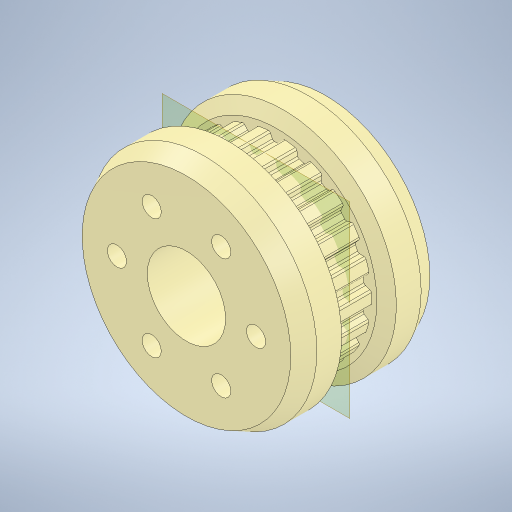
# Autodesk Inventor part: XL Pulley Generator
Saved by Autodesk Inventor 2023.4 (Build 274418000, 418)
## iProperties
RuleStatus: InUse
Created: 2022-06-22
Part Number: XL Pulley Generator
Material: Nylon 6/6
Document SubType Name: Modeling
Designer: Nathan Cai
Density: 1.13 g/cm^3
Appearance: Nylon 6
Mass: 3.49489 g
Surface Area: 67.8029 cm^2
Volume: 3.75794 cm^3
Author: Nathan Cai
Autodesk Inventor part; units mm, degrees
ref_plane "YZ Plane" through (0, 0, 0) normal (1, 0, 0) x (0, 1, 0)
ref_plane "XZ Plane" through (0, 0, 0) normal (0, 1, 0) x (-1, 0, 0)
ref_plane "XY Plane" through (0, 0, 0) normal (0, 0, 1) x (1, 0, 0)
sketch "Sketch2" plane through (0, 0, 0) normal (0, 0, 1) x (1, 0, 0)
  circle A0 centre (0, 0) radius 17.7872 construction
  circle A1 centre (0, 0) radius 17.2722
  dimension "Pd" = 35.5743
  dimension "OD" = 34.5443
  constraints: 2 centre point, 2 coincident
  measures "Pd" diameter of A0
  measures "OD" diameter of A1
extrude "Extrusion3" add sketch "Sketch2" along normal blind 7.62
sketch "Sketch3" plane through (0, 0, 7.62) normal (0, 0, 1) x (1, 0, 0)
  line L0 (0, 0) -> (0, 17.2722) construction
  circle A0 centre (0, 0) radius 17.2722 projected
  line L1 (0, 0) -> (4.8661, 16.5725) construction
  circle A1 centre (0, 0) radius 16.0022
  line L2 (0.8131, 16.2149) -> (1.172, 16.9846)
  line L3 (1.2838, 17.2244) -> (0, 0) construction
  arc A2 (1.5505, 17.2024) -> (1.172, 16.9846) centre (1.5164, 16.824) ccw
  arc A3 (0.4578, 15.9956) -> (0.8131, 16.2149) centre (0.4687, 16.3755) ccw
  circle A4 centre (0, 0) radius 17.2722 projected
  line L4 (-0.8131, 16.2149) -> (-1.172, 16.9846)
  arc A5 (-1.172, 16.9846) -> (-1.5505, 17.2024) centre (-1.5164, 16.824) ccw
  arc A6 (-0.8131, 16.2149) -> (-0.4578, 15.9956) centre (-0.4687, 16.3755) ccw
  point P0 (1.5692, 15.925)
  point P1 (1.5505, 17.2024)
  point P2 (-1.5505, 17.2024)
  point P3 (-0.4578, 15.9956)
  dimension "d29" = 16.364
  dimension "d30" = 32.0043
  dimension "d31" = 25
  dimension "d33" = 4.263
  dimension "d34" = 0.76
  dimension "d35" = 0.76
  constraints: 14 point on circle, 10 end point, 6 symmetric about line, 5 centre point, 4 tangent, 1 coincident, 1 point on line, 1 vertical, 2 other
  measures "d29" angle of L0 L1
  measures "d30" diameter of A1
  measures "d31" angle of L0 L2
  measures "d33" angle of L0 L3
  measures "d34" diameter of A2
  measures "d35" diameter of A3
extrude "Extrusion4" cut sketch "Sketch3" against normal through all contours A2 L2 A3 A1 A6 L4 A5 A0 picked at (-0.0509, 16.8435)
pattern_circular "Circular Pattern2" count 22 over 360 about axis through (0, 0, 0) along (0, 0, 1) of "Extrusion4"
ref_plane "Work Plane2" through (0, 0, 3.81) normal (0, 0, -1) x (-1, 0, 0)
sketch "Sketch5" plane through (0, 0, 7.62) normal (0, 0, 1) x (1, 0, 0)
  circle A0 centre (0, 0) radius 20.6375
  dimension "d48" = 41.275
  constraints: 1 centre point, 1 coincident
  measures "d48" diameter of A0
extrude "Extrusion6" add sketch "Sketch5" along normal blind 8.89
chamfer "Chamfer2" distance 1.1906 distance2 2.3813 1 edges at (-20.6375, 0, 7.62) measured on face at (20.5706, -1.6606, 13.5467)
chamfer "Chamfer3" distance 1.5875 distance2 3.175 1 edges at (-20.6375, 0, 16.51) measured on face at (6.6793, -1.6463, 16.51)
mirror "Mirror2" about plane through (0, 0, 3.81) normal (0, 0, -1) of "Extrusion6", "Chamfer2", "Chamfer3"
sketch "Sketch6" plane through (0, 0, -8.89) normal (0, 0, -1) x (-1, 0, 0)
  circle A0 centre (0, 0) radius 7.1437
  circle A1 centre (0, 0) radius 12.7 construction
  line L0 (0, 0) -> (12.7, 0) construction
  circle A2 centre (12.7, 0) radius 1.7526
  circle A3 centre (6.35, 10.9985) radius 1.7526
  circle A4 centre (-6.35, 10.9985) radius 1.7526
  circle A5 centre (-12.7, 0) radius 1.7526
  circle A6 centre (-6.35, -10.9985) radius 1.7526
  circle A7 centre (6.35, -10.9985) radius 1.7526
  dimension "d55" = 25.4
  dimension "d54" = 14.2875
  dimension "d56" = 3.5052
  dimension "d59" = 360
  constraints: 7 centre point, 3 coincident, 2 end point, 1 horizontal, 1 horizontal alignment, 15 other
  measures "d54" diameter of A0
  measures "d56" diameter of A2
extrude "Extrusion7" cut sketch "Sketch6" against normal through all
equation "\"pitch\" = 5.08"
equation "\"width\" = 7.62"
equation "\"T_angle\" = 50deg"
equation "\"T_ht\" = 1.27"
equation "\"r1\" = 0.38"
equation "\"r2\" = 0.38"
equation "\"T_hs\" = 2.3"
equation "\"T_s\" = 2.57"
body "Solid3"
